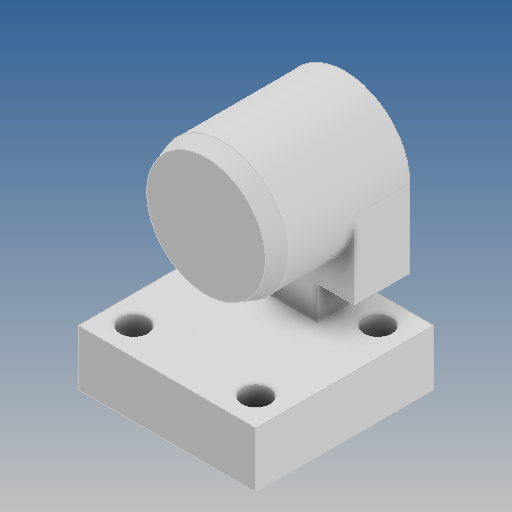
# Autodesk Inventor part: 0008-30-004
Saved by Autodesk Inventor 2020 (Build 240168000, 168)
## iProperties
Created: 2021-05-20
Part Number: 0008-30-004
Material: Generic
Document SubType Name: Modeling
Designer: Iulian Bors
Density: 1 g/cm^3
Appearance: Default
Author: Iulian Bors
Subject: 004
Autodesk Inventor part; units mm, degrees
ref_plane "YZ Plane" through (0, 0, 0) normal (1, 0, 0) x (0, 1, 0)
ref_plane "XZ Plane" through (0, 0, 0) normal (0, 1, 0) x (-1, 0, 0)
ref_plane "XY Plane" through (0, 0, 0) normal (0, 0, 1) x (1, 0, 0)
sketch "Sketch1" plane through (0, 0, 0) normal (0, 0, 1) x (1, 0, 0)
  circle A0 centre (0, 0) radius 11.7
  dimension "d0" = 23.4
  constraints: 1 centre point, 1 coincident
  measures "d0" diameter of A0
extrude "Extrusion1" add sketch "Sketch1" along normal blind 15
sketch "Sketch2" plane through (0, 0, 0) normal (0, 0, -1) x (-1, 0, 0)
  circle A0 centre (0, 0) radius 11.7 projected
  line L0 (-11.7, 0) -> (-11.7, -20)
  line L1 (-11.7, -20) -> (11.7, -20)
  line L2 (11.7, -20) -> (11.7, 0)
  circle A1 centre (0, 0) radius 11.7 projected
  line L3 (-11.7, 0) -> (11.7, 0)
  point P0 (11.7, 0)
  point P1 (-11.7, 0)
  dimension "d3" = 20
  constraints: 8 end point, 2 perpendicular, 2 point on circle, 2 tangent, 1 horizontal
  measures "d3" distance from line of L1 point (0, 0)
extrude "Extrusion2" add sketch "Sketch2" along normal blind 10
sketch "Sketch3" plane through (-11.7, -20, 0) normal (0, -1, 0) x (1, 0, 0)
  line L0 (-4.3, 22) -> (27.7, 22)
  line L1 (27.7, 22) -> (27.7, -10)
  line L2 (27.7, -10) -> (-4.3, -10)
  line L3 (-4.3, -10) -> (-4.3, 22)
  line L4 (23.4, -10) -> (0, -10) projected
  line L5 (23.4, 0) -> (0, 0) projected
  point P0 (11.7, 0)
  point P1 (11.7, 22)
  point P2 (11.7, 0)
  dimension "d6" = 32
  dimension "d7" = 32
  constraints: 8 end point, 2 midpoint, 2 parallel, 1 collinear, 1 horizontal, 1 perpendicular, 1 vertical alignment
  measures "d6" distance of L0.start L0.end
  measures "d7" distance of L2.end L0.start
extrude "Extrusion3" add sketch "Sketch3" along normal blind 10
sketch "Sketch4" plane through (-11.7, -30, 0) normal (0, -1, 0) x (1, 0, 0)
  line L0 (0.7, 17) -> (22.7, 17) construction
  line L1 (22.7, 17) -> (22.7, -5) construction
  line L2 (22.7, -5) -> (0.7, -5) construction
  line L3 (0.7, -5) -> (0.7, 17) construction
  line L4 (27.7, 22) -> (-4.3, 22) construction
  line L5 (-4.3, 22) -> (-4.3, -10) construction
  point P0 (11.7, 0)
  point P1 (11.7, 17)
  point P2 (11.7, 22)
  point P3 (0.7, 6)
  point P4 (-4.3, 6)
  dimension "d10" = 22
  dimension "d11" = 22
  constraints: 8 end point, 4 coincident, 4 midpoint, 2 parallel, 1 horizontal, 1 horizontal alignment, 1 perpendicular, 1 vertical alignment
  measures "d10" distance of L0.start L0.end
  measures "d11" distance of L0.end L1.end
hole "Hole1" at (-11, -30, 17) at (11, -30, 17) at (11, -30, -5) at (-11, -30, -5) direction (0, 1, 0) diameter 5 depth 10
sketch "Sketch5" plane through (0, 0, 0) normal (0, 0, 1) x (1, 0, 0)
  line L0 (11.7, -20) -> (-11.7, -20) projected
  line L1 (5, -20) -> (-5, -20)
  line L2 (-5, -20) -> (-5, -11.7)
  line L3 (-5, -11.7) -> (5, -11.7)
  line L4 (5, -11.7) -> (5, -20)
  circle A0 centre (0, 0) radius 11.7 projected
  line L5 (11.7, -20) -> (5, -20)
  line L6 (5, -20) -> (5, -14)
  line L7 (5, -14) -> (11.7, -14)
  line L8 (11.7, -14) -> (11.7, -20)
  line L9 (-5, -20) -> (-11.7, -20)
  line L10 (-11.7, -20) -> (-11.7, -14)
  line L11 (-11.7, -14) -> (-5, -14)
  line L12 (-5, -14) -> (-5, -20)
  line L13 (-11.7, -20) -> (-11.7, 0) projected
  line L14 (11.7, 0) -> (11.7, -20) projected
  point P0 (0, -11.7)
  dimension "d19" = 10
  dimension "d20" = 6
  constraints: 24 end point, 6 collinear, 6 parallel, 3 horizontal, 3 perpendicular, 2 point on line, 1 midpoint, 1 tangent, 1 vertical alignment
  measures "d19" distance between parallel lines of L2 L4
  measures "d20" distance of L7.end L5.start
extrude "Extrusion4" cut sketch "Sketch5" against normal through all contours L0 L4 L7 L8 | L0 L10 L11 L2
chamfer "Chamfer1" distance 1 distance2 3 1 edges at (-11.7, 0, 15) measured on face at (-1.2696, -2.7132, 15)
equation "\"d7\" = d6"
equation "\"d11\" = d10"
body "Solid1"
